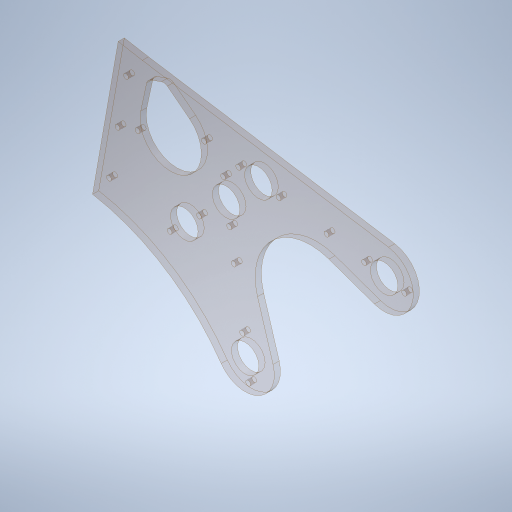
# Autodesk Inventor part: GP9-002
Saved by Autodesk Inventor 2023.4 (Build 274418000, 418)
## iProperties
Created: 2025-02-24
Part Number: GP9-002
Material: Polycarbonate, Smoke
Document SubType Name: Modeling
Designer: dlangdon
Density: 1.2 g/cm^3
Appearance: Polycarbonate - Smoked
Author: dlangdon
Autodesk Inventor part; units mm, degrees
ref_plane "YZ Plane" through (0, 0, 0) normal (1, 0, 0) x (0, 1, 0)
ref_plane "XZ Plane" through (0, 0, 0) normal (0, 1, 0) x (-1, 0, 0)
ref_plane "XY Plane" through (0, 0, 0) normal (0, 0, 1) x (1, 0, 0)
sketch "Sketch1" plane through (0, 0, 0) normal (0, 0, 1) x (1, 0, 0)
  circle A0 centre (71.842, 71.842) radius 50.8 construction
  circle A1 centre (-71.842, -71.842) radius 50.8 construction
  circle A2 centre (0, 0) radius 50.8 construction
  line L0 (-35.921, -35.921) -> (35.921, 35.921) construction
  line L1 (71.842, 71.842) -> (-71.842, -71.842) construction
  line L2 (-4.3707, 6.2419) -> (-4.3707, 50.6116) construction
  line L3 (-226.8798, -122.642) -> (638.5123, -122.642) construction
  circle A3 centre (147.8406, -65.492) radius 57.15 construction
  circle A4 centre (71.842, 71.842) radius 14.2875
  circle A5 centre (-71.842, -71.842) radius 14.2875
  circle A6 centre (-4.3707, 6.2419) radius 57.15 construction
  circle A7 centre (-71.842, -71.842) radius 30.1625 construction
  circle A8 centre (71.842, 71.842) radius 30.1625 construction
  circle A9 centre (-58.1587, 92.2793) radius 14.2875
  line L4 (-58.1587, 92.2793) -> (71.842, 71.842) construction
  circle A10 centre (71.842, 71.842) radius 14.3256 construction
  circle A11 centre (-71.842, -71.842) radius 14.3256 construction
  circle A12 centre (-91.5532, 58.2708) radius 14.2875
  line L5 (-71.842, -71.842) -> (-91.5532, 58.2708) construction
  circle A13 centre (-91.5532, 58.2708) radius 23.8316 construction
  circle A14 centre (-58.1587, 92.2793) radius 23.8316 construction
  line L6 (14.744, 60.1006) -> (61.7538, 43.4167)
  line L7 (-42.9911, -63.0445) -> (-59.0357, -10.4271)
  arc A15 (14.744, 60.1006) -> (-59.0357, -10.4271) centre (-4.3707, 6.2419) ccw
  line L8 (-203.1376, 146.1202) -> (-178.1235, 141.7096)
  line L9 (-178.1235, 141.7096) -> (-204.5875, -8.3751) construction
  line L10 (-204.5875, -8.3751) -> (-229.6016, -3.9645) construction
  line L11 (-229.6016, -3.9645) -> (-203.1376, 146.1202) construction
  line L12 (-245.2736, -92.8451) -> (35.0702, -142.2772) construction
  line L13 (-198.7269, 171.1343) -> (174.1389, 105.388) construction
  line L14 (-198.7269, 171.1343) -> (-245.2736, -92.8451) construction
  circle A16 centre (-148.7947, 88.6325) radius 31.75
  line L15 (-87.9836, 34.7081) -> (-79.4511, -21.6151) construction
  circle A17 centre (12.249, 81.2106) radius 9.525 construction
  line L16 (-190.6305, 143.9149) -> (-217.0945, -6.1698) construction
  line L17 (-195.0412, 118.9008) -> (-212.6839, 18.8443) construction
  circle A18 centre (-148.7947, 88.6325) radius 17.4625 construction
  circle A19 centre (-148.7947, 88.6325) radius 9.525
  circle A20 centre (-58.1587, 92.2793) radius 30.1816 construction
  line L18 (-203.1376, 146.1202) -> (-229.6016, -3.9645)
  arc A21 (61.7538, 43.4167) -> (76.5306, 101.6379) centre (71.842, 71.842) ccw
  arc A22 (-96.6164, -89.047) -> (-42.9911, -63.0445) centre (-71.842, -71.842) ccw
  line L19 (-148.7947, 88.6325) -> (-132.3853, 94.605) construction
  line L20 (-114.4841, 101.1205) -> (-183.1052, 76.1445) construction
  circle A23 centre (-183.1052, 76.1445) radius 4.7625 construction
  line L21 (0, 0) -> (-4.3707, 6.2419) construction
  circle A24 centre (71.842, 71.842) radius 28.6512 construction
  line L22 (64.3298, 44.1932) -> (-61.9049, 78.4917) construction
  line L23 (73.1757, 100.4622) -> (-57.4936, 106.5513) construction
  line L24 (-178.1235, 141.7096) -> (76.5306, 101.6379)
  line L25 (-148.7947, 88.6325) -> (-134.7687, 17.0965) construction
  circle A25 centre (-134.7687, 17.0965) radius 31.75 construction
  circle A26 centre (-134.7687, 17.0965) radius 14.2875
  line L26 (-91.5532, 58.2708) -> (-134.7687, 17.0965) construction
  circle A27 centre (-148.7947, 88.6325) radius 25.4 construction
  arc A28 (-96.6164, -89.047) -> (-229.6016, -3.9645) centre (-265.2541, -206.1602) ccw
  point P0 (-83.7173, 6.5465)
  point P1 (-203.8625, 68.8725)
  point P2 (-203.8625, 68.8725)
  point P3 (-145.7623, 105.8297)
  point P4 (-162.1717, 99.8571)
  point P5 (-165.204, 82.6599)
  point P6 (-151.827, 71.4353)
  point P7 (-135.4176, 77.4078)
  point P8 (-124.9265, 97.3198)
  point P9 (-144.384, 113.6466)
  point P10 (-168.2522, 104.9593)
  point P11 (-172.6629, 79.9452)
  point P12 (-153.2053, 63.6184)
  point P13 (-129.3371, 72.3057)
  dimension "d7" = 101.6
  dimension "d18" = 47.6631
  dimension "d34" = 34.925
  dimension "d65" = 50.8
  dimension "d3" = 45
  dimension "d4" = 0
  dimension "d8" = 101.6
  dimension "d9" = 28.575
  dimension "d10" = 101.6
  dimension "d11" = 114.3
  dimension "d12" = 114.3
  dimension "d13" = 15.875
  dimension "d14" = 15.875
  dimension "d15" = 131.5974
  dimension "d16" = 28.6512
  dimension "d17" = 131.5974
  dimension "d19" = 47.6631
  dimension "d22" = 25.4
  dimension "d23" = 152.4
  dimension "d26" = 268.0517
  dimension "d27" = 63.5
  dimension "d30" = 200.025
  dimension "d31" = 10
  dimension "d32" = 19.05
  dimension "d33" = 101.6
  dimension "d35" = 19.05
  dimension "d36" = 6.35
  dimension "d40" = 360
  dimension "d44" = 9.525
  dimension "d55" = 80
  dimension "d56" = 7.62
  dimension "d57" = 25.4
  dimension "d58" = 57.3024
  dimension "d59" = 63.5
  dimension "d60" = 72.898
  dimension "d61" = 59.69
  dimension "d62" = 55
  dimension "d68" = 360
  dimension "d70" = 38.1
  dimension "d71" = 60
  constraints: 54 end point, 25 centre point, 23 coincident, 21 point on circle, 16 tangent, 7 midpoint, 6 equal radius, 5 point on line, 4 collinear, 4 parallel, 2 horizontal, 1 concentric, 1 perpendicular, 1 vertical, 29 other
  measures "d3" angle of L2 L0
  measures "d4" distance between parallel lines of L0 L1
  measures "d8" diameter of A2
  measures "d9" diameter of A4
  measures "d10" diameter of A0
  measures "d11" diameter of A3
  measures "d12" diameter of A6
  measures "d13" radial gap between concentric circles of A5 A7
  measures "d14" radial gap between concentric circles of A4 A8
  measures "d15" distance of L4.start L4.end
  measures "d16" diameter of A10
  measures "d17" distance of L5.start L5.end
  measures "d19" diameter of A14
  measures "d22" distance of L9.end L10.end
  measures "d23" distance of L10.end L8.start
  measures "d26" distance of L13.start L12.start
  measures "d27" diameter of A16
  measures "d30" distance from line of point (0, 0) L9
  measures "d31" angle of L3 L12
  measures "d32" diameter of A17
  measures "d33" distance of L17.start L17.end
  measures "d35" diameter of A19
  measures "d36" radial gap between concentric circles of A14 A20
  measures "d44" diameter of A23
  measures "d55" angle of L1 L21
  measures "d56" distance of L21.start L21.end
  measures "d57" distance between parallel lines of L13 L8
  measures "d58" diameter of A24
  measures "d59" diameter of A25
  measures "d60" distance of L19.start L25.end
  measures "d61" distance of L26.start L26.end
  measures "d62" angle of L15 L26
  measures "d70" distance from line of L9 L19.start
  measures "d71" angle of L9 L20
extrude "Extrusion1" add sketch "Sketch1" along normal blind 6.35 contours A15 L7 A22 A28 L18 L8 L24 A21 L6
hole "Hole1" at (12.249, 81.2106, 0) at (-195.0412, 118.9008, 0) at (-203.8625, 68.8725, 0) at (-212.6839, 18.8443, 0) at (-132.3853, 94.605, 0) at (-145.7623, 105.8297, 0) at (-162.1717, 99.8571, 0) at (-165.204, 82.6599, 0) at (-151.827, 71.4353, 0) at (-135.4176, 77.4078, 0) at (-114.4841, 101.1205, 0) at (-183.1052, 76.1445, 0) at (-153.2053, 63.6184, 0) at (-172.6629, 79.9452, 0) at (-168.2522, 104.9593, 0) at (-144.384, 113.6466, 0) at (-124.9265, 97.3198, 0) at (-129.3371, 72.3057, 0) at (-83.7173, 6.5465, 0) direction (0, 0, 1) diameter 5.1054 end through all clearance for "Flat Head Machine Screw (82)" size "#10" standard "Ansi Unified Screw Threads"
sketch "Sketch2" plane through (0, 0, 6.35) normal (0, 0, 1) x (1, 0, 0)
  circle A0 centre (-183.1052, 76.1445) radius 2.5527 construction
  circle A1 centre (-212.6839, 18.8443) radius 2.5527 construction
  circle A2 centre (-195.0412, 118.9008) radius 2.5527 construction
  circle A3 centre (12.249, 81.2106) radius 2.5527 construction
  circle A4 centre (-203.8625, 68.8725) radius 2.5527 construction
  circle A5 centre (-114.4841, 101.1205) radius 2.5527 construction
  circle A6 centre (-83.7173, 6.5465) radius 2.5527 construction
  line L0 (-42.9911, -63.0445) -> (-59.0357, -10.4271) construction
  arc A7 (14.744, 60.1006) -> (-59.0357, -10.4271) centre (-4.3707, 6.2419) ccw construction
  line L1 (14.744, 60.1006) -> (61.7538, 43.4167) construction
  arc A8 (61.7538, 43.4167) -> (76.5306, 101.6379) centre (71.842, 71.842) ccw construction
  line L2 (76.5306, 101.6379) -> (-178.1235, 141.7096) construction
  line L3 (-178.1235, 141.7096) -> (-203.1376, 146.1202) construction
  line L4 (-203.1376, 146.1202) -> (-229.6016, -3.9645) construction
  arc A9 (-96.6164, -89.047) -> (-229.6016, -3.9645) centre (-265.2541, -206.1602) ccw construction
  arc A10 (-96.6164, -89.047) -> (-42.9911, -63.0445) centre (-71.842, -71.842) ccw construction
  circle A11 centre (-91.5532, 58.2708) radius 14.2875 construction
  circle A12 centre (-134.7687, 17.0965) radius 14.2875 construction
  circle A13 centre (-58.1587, 92.2793) radius 14.2875 construction
  circle A14 centre (-71.842, -71.842) radius 14.2875 construction
  circle A15 centre (71.842, 71.842) radius 14.2875 construction
  line L5 (-74.9903, -51.0607) -> (-68.6938, -92.6234) construction
  line L6 (-149.986, 2.5979) -> (-119.5513, 31.5951) construction
  line L7 (-94.7014, 79.0522) -> (-88.4049, 37.4894) construction
  line L8 (-78.9222, 95.5435) -> (-37.3952, 89.0151) construction
  line L9 (51.0786, 75.1063) -> (92.6055, 68.5778) construction
  circle A16 centre (-91.5532, 58.2708) radius 14.2875 construction
  line L10 (-58.1587, 92.2793) -> (-91.5532, 58.2708) construction
  line L11 (-58.1587, 92.2793) -> (71.842, 71.842) construction
  line L12 (-91.5532, 58.2708) -> (-134.7687, 17.0965) construction
  line L13 (-91.5532, 58.2708) -> (-71.842, -71.842) construction
  point P0 (0, 0)
  dimension "d72" = 42.037
  constraints: 19 end point, 14 coincident, 5 collinear, 5 midpoint, 4 equal length
  measures "d72" distance of L5.start L5.end
hole "Hole2" at (-74.9903, -51.0607, 6.35) at (-119.5513, 31.5951, 6.35) at (-68.6938, -92.6234, 6.35) at (-149.986, 2.5979, 6.35) at (-88.4049, 37.4894, 6.35) at (-94.7014, 79.0522, 6.35) at (-37.3952, 89.0151, 6.35) at (-78.9222, 95.5435, 6.35) at (92.6055, 68.5778, 6.35) at (51.0786, 75.1063, 6.35) direction (0, 0, -1) diameter 5.1054 end through all clearance for "Flat Head Machine Screw (82)" size "#10" standard "Ansi Unified Screw Threads"
sketch "Sketch3" plane through (0, 0, 6.35) normal (0, 0, 1) x (1, 0, 0)
  circle A0 centre (-148.7947, 88.6325) radius 31.75 projected
  line L0 (-179.8269, 95.3455) -> (-172.948, 127.1441)
  line L1 (-172.948, 127.1441) -> (-155.0469, 133.6595)
  line L2 (-155.0469, 133.6595) -> (-129.3377, 113.7221)
  circle A1 centre (-114.4841, 101.1205) radius 2.5527 projected
  circle A2 centre (-183.1052, 76.1445) radius 2.5527 projected
  line L3 (-114.4841, 101.1205) -> (-183.1052, 76.1445) construction
  line L4 (-183.1052, 76.1445) -> (-148.7947, 88.6325)
  line L5 (-148.7947, 88.6325) -> (-163.9975, 130.4018) construction
  point P0 (0, 0)
  dimension "d80" = 44.45
  dimension "d82" = 19.05
  constraints: 12 end point, 2 point on circle, 2 tangent, 1 collinear, 1 equal length, 1 midpoint, 1 perpendicular
  measures "d80" distance from line of L4.end L1
  measures "d82" distance of L0.end L1.end
extrude "Extrusion2" cut sketch "Sketch3" against normal through all contours A0 L0 L1 L2
fillet "Fillet1" radius 6.35 2 edges at (-172.948, 127.1441, 3.175) (-155.0469, 133.6595, 3.175)
body "Solid1"
